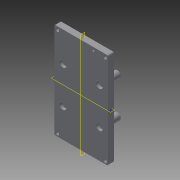
# Autodesk Inventor part: porte_carte
Saved by Autodesk Inventor 2015 (Build 190159000, 159)
## iProperties
Created: 2015-02-17
Part Number: porte_carte
Material: Generic
Document SubType Name: Modeling
Designer: Piotr
Density: 1 g/cm^3
Appearance: Default
Author: Piotr
Autodesk Inventor part; units mm, degrees
ref_plane "YZ Plane" through (0, 0, 0) normal (1, 0, 0) x (0, 1, 0)
ref_plane "XZ Plane" through (0, 0, 0) normal (0, 1, 0) x (-1, 0, 0)
ref_plane "XY Plane" through (0, 0, 0) normal (0, 0, 1) x (1, 0, 0)
sketch "Sketch1" plane through (0, 0, 0) normal (0, 1, 0) x (-1, 0, 0)
  line L0 (-22.5, 40) -> (22.5, 40)
  line L1 (22.5, 40) -> (22.5, -40)
  line L2 (22.5, -40) -> (-22.5, -40)
  line L3 (-22.5, -40) -> (-22.5, 40)
  line L4 (-22.5, 40) -> (22.5, -40) construction
  line L5 (22.5, 40) -> (-22.5, -40) construction
  point P0 (0, 0)
  dimension "d0" = 80
  dimension "d1" = 45
  constraints: 12 end point, 2 midpoint, 2 parallel, 1 horizontal, 1 perpendicular
  measures "d0" distance of L0.end L1.end
  measures "d1" distance of L1.end L2.end
extrude "Extrusion1" add sketch "Sketch1" along normal blind 5
ref_plane "Work Plane1" through (22.5, 0, 0) normal (0, 0, -1) x (-1, 0, 0)
ref_plane "Work Plane2" through (0, 0, 40) normal (1, 0, 0) x (0, 0, -1)
sketch "Sketch2" plane through (0, 5, 0) normal (0, 1, 0) x (1, 0, 0)
  line L0 (-22.5, 40) -> (22.5, 40) projected
  line L1 (22.5, -40) -> (22.5, 40) projected
  point P0 (0, 0)
  point P1 (20, 37.5)
  dimension "d4" = 2.5
  dimension "d5" = 2.5
  measures "d4" distance from line of L0 point (20, 37.5)
  measures "d5" distance from line of L1 point (20, 37.5)
hole "Hole1" at (20, 5, -37.5) direction (0, -1, 0) diameter 3.1 end through all
fillet "Fillet1" radius 1 1 edges at (22.5, 2.5, -40)
sketch "Sketch3" plane through (0, 5, 0) normal (0, 1, 0) x (1, 0, 0)
  circle A0 centre (15.25, 15.25) radius 3
  line L0 (-31.5, 0) -> (31.5, 0) construction
  line L1 (0, 56) -> (0, -56) construction
  point P0 (0, 0)
  dimension "d14" = 15.25
  dimension "d15" = 15.25
  dimension "d16" = 6
  constraints: 1 centre point
  measures "d14" distance from line of A0.centre L0
  measures "d15" distance from line of L1 A0.centre
  measures "d16" diameter of A0
extrude "Extrusion2" add sketch "Sketch3" along normal blind 10
hole "Hole2" at (15.25, 15, -15.25) direction (0, -1, 0) diameter 3.1 depth 11 tip angle 118
sketch "Sketch5" plane through (0, 0, 0) normal (0, -1, 0) x (1, 0, 0)
  circle A0 centre (15.25, -15.25) radius 3 projected
  point P0 (0, 0)
extrude "Extrusion3" cut sketch "Sketch5" against normal blind 2.3
fillet "Fillet2" radius 3 1 edges at (12.25, 5, -15.25)
mirror "Mirror1" about plane through (0, 0, 40) normal (1, 0, 0) of "Hole2", "Extrusion2", "Fillet1", "Hole1", "Extrusion3", "Fillet2"
mirror "Mirror2" about plane through (22.5, 0, 0) normal (0, 0, -1) of "Hole2", "Extrusion2", "Fillet1", "Hole1", "Mirror1", "Extrusion3", "Fillet2"
sketch "Sketch4" plane through (0, 5, 0) normal (0, 1, 0) x (1, 0, 0)
  circle A0 centre (-20, -37.5) radius 1.55 construction
  line L0 (-21.5, -40) -> (21.5, -40) construction
  point P0 (0, 0)
  point P1 (10, -37.5)
  dimension "d30" = 30
  measures "d30" distance of point (10, -37.5) A0.centre
hole "Hole3" at (10, 5, 37.5) direction (0, -1, 0) diameter 2 end through all
equation "\"d14\" = d15"
body "Solid1"
